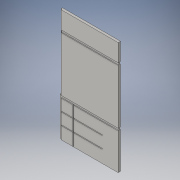
# Autodesk Inventor part: Vertical Shelf cut short (2.3.2018)
Saved by Autodesk Inventor 2016 (Build 200138000, 138)
## iProperties
Created: 2017-10-31
Part Number: Vertical Shelf cut short (2.3.2018)
Material: Generic
Document SubType Name: Modeling
Designer: mathaetaes
Density: 1 g/cm^3
Appearance: Default
Author: mathaetaes
Autodesk Inventor part; units mm, degrees
ref_plane "YZ Plane" through (0, 0, 0) normal (1, 0, 0) x (0, 1, 0)
ref_plane "XZ Plane" through (0, 0, 0) normal (0, 1, 0) x (-1, 0, 0)
ref_plane "XY Plane" through (0, 0, 0) normal (0, 0, 1) x (1, 0, 0)
sketch "Sketch1" plane through (0, 0, 0) normal (0, 0, 1) x (1, 0, 0)
  line L0 (-185.0798, 623.3432) -> (284.8202, 623.3432)
  line L1 (284.8202, 623.3432) -> (284.8202, -278.3568)
  line L2 (284.8202, -278.3568) -> (-185.0798, -278.3568)
  line L3 (-185.0798, -278.3568) -> (-185.0798, 623.3432)
  point P0 (0, 0)
  dimension "d0" = 901.7
  dimension "d1" = 469.9
  constraints: 8 end point, 2 parallel, 1 horizontal, 1 perpendicular
  measures "d0" distance of L0.end L1.end
  measures "d1" distance of L1.end L2.end
extrude "Board" add sketch "Sketch1" along normal blind 19.05
sketch "Sketch6" plane through (0, 0, 0) normal (0, 0, -1) x (-1, 0, 0)
  line L0 (-284.8202, 483.6432) -> (185.0798, 483.6432)
  line L1 (185.0798, 483.6432) -> (185.0798, 464.5932)
  line L2 (185.0798, 464.5932) -> (-284.8202, 464.5932)
  line L3 (-284.8202, 464.5932) -> (-284.8202, 483.6432)
  line L4 (185.0798, 623.3432) -> (-284.8202, 623.3432) projected
  line L5 (185.0798, -278.3568) -> (185.0798, 623.3432) projected
  line L6 (-284.8202, 623.3432) -> (-284.8202, -278.3568) projected
  line L7 (-284.8202, 29.6182) -> (185.0798, 29.6182)
  line L8 (185.0798, 29.6182) -> (185.0798, 10.5682)
  line L9 (185.0798, 10.5682) -> (-284.8202, 10.5682)
  line L10 (-284.8202, 10.5682) -> (-284.8202, 29.6182)
  point P0 (0, 0)
  dimension "d30" = 19.05
  dimension "d37" = 434.975
  dimension "d119" = 139.7
  constraints: 16 end point, 5 collinear, 4 parallel, 2 horizontal, 2 perpendicular
  measures "d30" distance of L0.end L1.end
  measures "d37" distance between parallel lines of L7 L2
  measures "d119" distance between parallel lines of L4 L0
extrude "Right Shelf Dados" cut sketch "Sketch6" against normal blind 6.35 contours L0 L1 L2 L3 | L7 L5 L9 L6
sketch "Sketch32" plane through (0, 0, 0) normal (0, 0, -1) x (-1, 0, 0)
  line L0 (-157.8202, -78.3318) -> (185.0798, -78.3318)
  line L1 (185.0798, -78.3318) -> (185.0798, -84.6818)
  line L2 (185.0798, -84.6818) -> (-157.8202, -84.6818)
  line L3 (-157.8202, -84.6818) -> (-157.8202, -78.3318)
  line L4 (-157.8202, -173.5818) -> (185.0798, -173.5818)
  line L5 (185.0798, -173.5818) -> (185.0798, -179.9318)
  line L6 (185.0798, -179.9318) -> (-157.8202, -179.9318)
  line L7 (-157.8202, -179.9318) -> (-157.8202, -173.5818)
  line L8 (-284.8202, 623.3432) -> (-284.8202, -278.3568) projected
  line L9 (185.0798, 623.3432) -> (185.0798, -278.3568) projected
  line L10 (-284.8202, -278.3568) -> (185.0798, -278.3568) projected
  point P0 (0, 0)
  point P1 (-284.8202, 10.5682)
  dimension "d142" = 88.9
  dimension "d143" = 6.35
  dimension "d146" = 342.9
  dimension "d167" = 127
  dimension "d170" = 98.425
  constraints: 16 end point, 4 parallel, 3 collinear, 2 horizontal, 2 perpendicular, 1 point on line
  measures "d142" distance between parallel lines of L2 L4
  measures "d143" distance between parallel lines of L0 L2
  measures "d146" distance of L1.end L2.end
  measures "d167" distance between parallel lines of L3 L8
  measures "d170" distance between parallel lines of L10 L6
extrude "Right Wine Rack Horizonal Dados" cut sketch "Sketch32" against normal blind 6.35
sketch "Sketch33" plane through (0, 0, 0) normal (0, 0, -1) x (-1, 0, 0)
  line L0 (185.0798, 10.5682) -> (-284.8202, 10.5682) projected
  line L1 (70.7798, 10.5682) -> (77.1298, 10.5682)
  line L2 (77.1298, 10.5682) -> (77.1298, -278.3568)
  line L3 (77.1298, -278.3568) -> (70.7798, -278.3568)
  line L4 (70.7798, -278.3568) -> (70.7798, 10.5682)
  line L5 (-157.8202, -84.6818) -> (-157.8202, -78.3318) projected
  line L6 (-284.8202, -278.3568) -> (185.0798, -278.3568) projected
  point P0 (0, 0)
  dimension "d149" = 6.35
  dimension "d168" = 228.6
  constraints: 8 end point, 2 parallel, 1 collinear, 1 horizontal, 1 perpendicular, 1 point on line
  measures "d149" distance between parallel lines of L2 L4
  measures "d168" distance between parallel lines of L5 L4
extrude "Right Wine Rack Vertical Dado" cut sketch "Sketch33" against normal blind 6.35
sketch "Sketch7" plane through (0, 0, 19.05) normal (0, 0, 1) x (1, 0, 0)
  line L0 (-185.0798, 483.6432) -> (284.8202, 483.6432)
  line L1 (284.8202, 483.6432) -> (284.8202, 464.5932)
  line L2 (284.8202, 464.5932) -> (-185.0798, 464.5932)
  line L3 (-185.0798, 464.5932) -> (-185.0798, 483.6432)
  line L4 (284.8202, 483.6432) -> (-185.0798, 483.6432) projected
  line L5 (-185.0798, 464.5932) -> (284.8202, 464.5932) projected
  line L6 (284.8202, -278.3568) -> (284.8202, 623.3432) projected
  line L7 (-185.0798, 623.3432) -> (-185.0798, -278.3568) projected
  line L8 (-185.0798, 29.6182) -> (284.8202, 29.6182)
  line L9 (284.8202, 29.6182) -> (284.8202, 10.5682)
  line L10 (284.8202, 10.5682) -> (-185.0798, 10.5682)
  line L11 (-185.0798, 10.5682) -> (-185.0798, 29.6182)
  point P0 (0, 0)
  point P1 (284.8202, 20.0932)
  dimension "d36" = 434.975
  constraints: 16 end point, 7 collinear, 4 parallel, 2 horizontal, 2 perpendicular
  measures "d36" distance between parallel lines of L8 L2
extrude "Left Shelf Dados" cut sketch "Sketch7" against normal blind 6.35 contours L0 L1 L2 L3 | L8 L6 L10 L7
sketch "Sketch34" plane through (0, 0, 19.05) normal (0, 0, 1) x (1, 0, 0)
  line L0 (157.8202, -78.3318) -> (-185.0798, -78.3318)
  line L1 (-185.0798, -78.3318) -> (-185.0798, -84.6818)
  line L2 (-185.0798, -84.6818) -> (157.8202, -84.6818)
  line L3 (157.8202, -84.6818) -> (157.8202, -78.3318)
  line L4 (157.8202, -173.5818) -> (-185.0798, -173.5818)
  line L5 (-185.0798, -173.5818) -> (-185.0798, -179.9318)
  line L6 (-185.0798, -179.9318) -> (157.8202, -179.9318)
  line L7 (157.8202, -179.9318) -> (157.8202, -173.5818)
  line L8 (284.8202, -278.3568) -> (284.8202, 10.5682) projected
  line L9 (-185.0798, 10.5682) -> (-185.0798, 483.6432) projected
  line L10 (-185.0798, -278.3568) -> (284.8202, -278.3568) projected
  point P0 (0, 0)
  dimension "d153" = 6.35
  dimension "d155" = 88.9
  dimension "d164" = 127
  dimension "d171" = 98.425
  constraints: 16 end point, 4 parallel, 3 collinear, 2 horizontal, 2 perpendicular, 1 point on line
  measures "d153" distance between parallel lines of L0 L2
  measures "d155" distance between parallel lines of L2 L4
  measures "d164" distance between parallel lines of L8 L3
  measures "d171" distance between parallel lines of L10 L6
extrude "Left Wine Rack Horizontal Dados" cut sketch "Sketch34" against normal blind 6.35
sketch "Sketch35" plane through (0, 0, 19.05) normal (0, 0, 1) x (1, 0, 0)
  line L0 (284.8202, 10.5682) -> (-185.0798, 10.5682) projected
  line L1 (-77.1298, 10.5682) -> (-70.7798, 10.5682)
  line L2 (-70.7798, 10.5682) -> (-70.7798, -278.3568)
  line L3 (-70.7798, -278.3568) -> (-77.1298, -278.3568)
  line L4 (-77.1298, -278.3568) -> (-77.1298, 10.5682)
  line L5 (157.8202, -78.3318) -> (157.8202, -84.6818) projected
  line L6 (-185.0798, -278.3568) -> (284.8202, -278.3568) projected
  point P0 (0, 0)
  dimension "d159" = 6.35
  dimension "d165" = 228.6
  constraints: 8 end point, 2 parallel, 1 collinear, 1 horizontal, 1 perpendicular, 1 point on line
  measures "d159" distance between parallel lines of L2 L4
  measures "d165" distance between parallel lines of L5 L2
extrude "Left Wine Rack  Vertical Dado" cut sketch "Sketch35" against normal blind 6.35
sketch "Sketch10" plane through (0, 0, 19.05) normal (0, 0, 1) x (1, 0, 0)
  line L0 (284.8202, -278.3568) -> (-185.0798, -278.3568) projected
  line L1 (-185.0798, 623.3432) -> (-172.3798, 623.3432)
  line L2 (-172.3798, 623.3432) -> (-172.3798, -278.3568)
  line L3 (-172.3798, -278.3568) -> (-185.0798, -278.3568)
  line L4 (-185.0798, -278.3568) -> (-185.0798, 623.3432)
  point P0 (0, 0)
  point P1 (-77.1298, -278.3568)
  dimension "d48" = 12.7
  constraints: 8 end point, 2 parallel, 1 horizontal, 1 perpendicular, 1 point on line
  measures "d48" distance between parallel lines of L4 L2
extrude "Vertical Wire Channel" cut sketch "Sketch10" against normal blind 6.35
sketch "Sketch12" plane through (-185.0798, -278.3568, 12.7) normal (-1, 0, 0) x (0, 0, 1)
  line L0 (-6.35, 742.95) -> (0, 742.95)
  line L1 (0, 742.95) -> (0, 749.3)
  line L2 (0, 749.3) -> (-6.35, 749.3)
  line L3 (-6.35, 749.3) -> (-6.35, 742.95)
  line L4 (0, 0) -> (0, 901.7) projected
  line L5 (-6.35, 742.95) -> (-12.7, 742.95) projected
  dimension "d51" = 6.35
  constraints: 8 end point, 2 collinear, 2 parallel, 1 coincident, 1 horizontal, 1 perpendicular
  measures "d51" distance between parallel lines of L2 L0
extrude "Top Horizontal Wire Channel" cut sketch "Sketch12" against normal blind 12.7
sketch "Sketch20" plane through (0, 0, 0) normal (0, 0, -1) x (-1, 0, 0)
  line L0 (185.0798, 623.3432) -> (-284.8202, 623.3432) projected
  line L1 (-284.8202, 29.6182) -> (185.0798, 29.6182) projected
  line L2 (185.0798, 623.3432) -> (178.7298, 623.3432)
  line L3 (178.7298, 623.3432) -> (178.7298, 29.6182)
  line L4 (178.7298, 29.6182) -> (185.0798, 29.6182)
  line L5 (185.0798, 29.6182) -> (185.0798, 623.3432)
  point P0 (0, 0)
  dimension "d99" = 6.35
  constraints: 8 end point, 2 parallel, 1 horizontal, 1 perpendicular, 1 point on line
  measures "d99" distance of L4.end L3.end
extrude "Rear Top Panel Dado" cut sketch "Sketch20" against normal blind 12.7
sketch "Sketch21" plane through (-185.0798, -278.3568, 0) normal (-1, 0, 0) x (0, 0, 1)
  line L0 (0, 200.025) -> (0, 288.925) projected
  line L1 (0, 288.925) -> (6.35, 288.925)
  line L2 (6.35, 288.925) -> (6.35, 0)
  line L3 (0, 0) -> (0, 288.925)
  line L4 (0, 0) -> (6.35, 0)
  line L5 (0, 0) -> (12.7, 0) projected
  constraints: 8 end point, 2 horizontal, 1 collinear, 1 parallel, 1 perpendicular
extrude "Bottom Panel Dado" cut sketch "Sketch21" against normal blind 6.35
body "Solid1"
